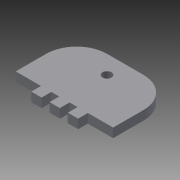
# Autodesk Inventor part: link1
Saved by Autodesk Inventor 2014 SP1 (Build 180222100, 222)
## iProperties
Created: 2015-02-17
Part Number: link1
Material: Generic
Document SubType Name: Modeling
Designer: Erin
Density: 1 g/cm^3
Appearance: Default
Author: Erin
Autodesk Inventor part; units mm, degrees
ref_plane "YZ Plane" through (0, 0, 0) normal (1, 0, 0) x (0, 1, 0)
ref_plane "XZ Plane" through (0, 0, 0) normal (0, 1, 0) x (-1, 0, 0)
ref_plane "XY Plane" through (0, 0, 0) normal (0, 0, 1) x (1, 0, 0)
sketch "tabs" plane through (0, 0, 0) normal (0, 0, 1) x (1, 0, 0)
  line L0 (15.6175, 13.9118) -> (18.7675, 13.9118)
  line L1 (18.7675, 13.9118) -> (18.7675, 10.7868)
  line L2 (18.7675, 10.7868) -> (15.6175, 10.7868)
  line L3 (15.6175, 10.7868) -> (15.6175, 13.9118)
  line L4 (21.8175, 13.9118) -> (24.9675, 13.9118)
  line L5 (24.9675, 13.9118) -> (24.9675, 10.7868)
  line L6 (24.9675, 10.7868) -> (21.8175, 10.7868)
  line L7 (21.8175, 10.7868) -> (21.8175, 13.9118)
  line L8 (28.0175, 13.9118) -> (31.1675, 13.9118)
  line L9 (31.1675, 13.9118) -> (31.1675, 10.7868)
  line L10 (31.1675, 10.7868) -> (28.0175, 10.7868)
  line L11 (28.0175, 10.7868) -> (28.0175, 13.9118)
  line L12 (23.3925, 10.7868) -> (23.3925, 8.8536) construction
  point P0 (23.3925, 12.1901)
  dimension "d2" = 3.15
  dimension "d3" = 3.05
  dimension "d4" = 3.05
  dimension "d5" = 3.125
  measures "d2" distance of L1.end L2.end
  measures "d3" distance between parallel lines of L7 L1
  measures "d4" distance between parallel lines of L11 L5
  measures "d5" distance of L2.end L0.start
sketch "Sketch1" plane through (0, 0, 0) normal (0, 0, 1) x (1, 0, 0)
  line L0 (-6, 20) -> (6, 20)
  line L1 (16, 10) -> (16, 0)
  line L2 (16, 0) -> (-16, 0)
  line L3 (-16, 0) -> (-16, 10)
  line L4 (0, 16.9043) -> (0, -20.0235) construction
  line L5 (-32.3473, 0) -> (40.4078, 0) construction
  arc A0 (-6, 20) -> (-16, 10) centre (-6, 10) ccw
  arc A1 (16, 10) -> (6, 20) centre (6, 10) ccw
  circle A2 centre (0, 14) radius 1.5
  line L6 (-7.775, 0) -> (-4.625, 0)
  line L7 (-4.625, 0) -> (-4.625, -3.125)
  line L8 (-4.625, -3.125) -> (-7.775, -3.125)
  line L9 (-7.775, -3.125) -> (-7.775, 0)
  line L10 (-1.575, 0) -> (1.575, 0)
  line L11 (1.575, 0) -> (1.575, -3.125)
  line L12 (1.575, -3.125) -> (-1.575, -3.125)
  line L13 (-1.575, -3.125) -> (-1.575, 0)
  line L14 (4.625, 0) -> (7.775, 0)
  line L15 (7.775, 0) -> (7.775, -3.125)
  line L16 (7.775, -3.125) -> (4.625, -3.125)
  line L17 (4.625, -3.125) -> (4.625, 0)
  line L18 (0, -3.125) -> (0, -5.0582) construction
  point P0 (0, 0)
  point P1 (0, 20)
  point P2 (16, 5)
  dimension "d0" = 32
  dimension "d6" = 20
  dimension "d7" = 10
  dimension "d8" = 3
  dimension "d9" = 6
  constraints: 12 end point, 4 point on circle, 4 tangent, 3 centre point, 3 horizontal, 3 parallel, 2 midpoint, 2 perpendicular, 2 vertical, 1 collinear, 1 equal radius, 1 point on line, 1 vertical alignment
  measures "d0" distance of L1.end L2.end
  measures "d6" distance between parallel lines of L2 L0
  measures "d7" radius of A0
  measures "d8" diameter of A2
  measures "d9" distance from line of A2.centre L0
extrude "Extrusion1" add sketch "Sketch1" along normal blind 3.1
equation "\"d2\" = mat + kerf"
equation "\"d3\" = mat - kerf"
equation "\"d4\" = mat - kerf"
equation "\"d5\" = mat + 0.5 * kerf"
equation "\"d10\" = mat"
equation "\"mat\" = 3.1"
equation "\"kerf\" = 0.05"
body "Solid1"
